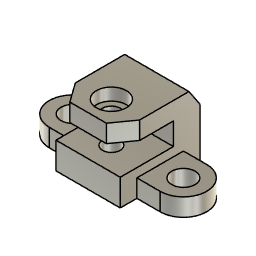
exercise05 (Autodesk Fusion 360 design; units mm, degrees)
Autodesk Fusion 360 part; units mm, degrees
sketch "草图1" plane through (0, 0, 0) normal (0, 0, 1) x (1, 0, 0)
  line L0 (-125, 0) -> (125, 0) construction
  line L1 (0, -50) -> (0, 50) construction
  line L2 (-58, 0) -> (58, 0)
  line L3 (58, 30) -> (58, 0)
  line L4 (58, 30) -> (100, 30)
  line L5 (-58, 0) -> (-58, 30)
  line L6 (-58, 30) -> (-100, 30)
  circle A0 centre (-100, 72) radius 21
  circle A1 centre (100, 72) radius 21
  circle A2 centre (0, 42) radius 16
  line L7 (-100, 114) -> (-58, 114)
  line L8 (-58, 114) -> (-58, 144)
  line L9 (-58, 144) -> (58, 144)
  line L10 (58, 144) -> (58, 114)
  line L11 (58, 114) -> (100, 114)
  arc A3 (100, 30) -> (100, 114) centre (100, 72) ccw
  arc A4 (-100, 114) -> (-100, 30) centre (-100, 72) ccw
  line L12 (-58, 114) -> (-58, 30)
  line L13 (58, 114) -> (58, 30)
  dimension "d1" = 116
  dimension "d2" = 144
  dimension "d3" = 72
  dimension "d4" = 200
  dimension "d5" = 84
  dimension "d6" = 42
  dimension "d7" = 32
  dimension "d8" = 42
  constraint horizontal L0
  constraint vertical L1
  constraint coincident L0 L2.start
  constraint coincident L0 L2.end
  constraint perpendicular L0 L3
  constraint perpendicular L3 L4
  constraint perpendicular L2 L5
  constraint perpendicular L5 L6
  constraint concentric A0 A4
  constraint concentric A1 A3
  constraint vertical L8
  constraint perpendicular L8 L9
  constraint perpendicular L8 L11
  constraint equal A3 A4
  constraint equal A0 A1
  constraint parallel L0 L7
  constraint perpendicular L9 L10
  constraint symmetric L1 L8 L10
  constraint symmetric L1 L3 L5
  constraint equal L3 L5
  constraint equal L8 L10
  constraint symmetric L1 A0.centre A1.centre
  constraint collinear L1.start L1.end A2.centre
  constraint tangent L4 A4
  constraint tangent L7 A4
  constraint collinear L5 L8
  measures "d1" distance of L2.start L2.end
  measures "d2" vertical distance of L2.end L9.end
  measures "d3" vertical distance of A1.centre L9.end
  measures "d4" distance of A0.centre A1.centre
  measures "d5" diameter of A3
  measures "d6" diameter of A1
  measures "d7" diameter of A2
  measures "d8" distance of L2 A2.centre
extrude "拉伸1" add sketch "草图1" along normal blind 32 contours L6 L7 A4 L12 | L4 L11 A3 L13 makes body 1 at (65, 72, 0) makes body 2 at (-65, 72, 0)
extrude "拉伸2" add sketch "草图1" along normal blind 48 contours L2 L3 L5 L8 L9 L10 L12 L13 bodies 1 2
sketch "草图2" plane through (-58, 0, 0) normal (-1, 0, 0) x (0, -1, 0)
  line L0 (-114, 0) -> (-114, 32)
  line L1 (-114, 32) -> (-30, 32)
  line L2 (-30, 32) -> (-30, 0)
  line L3 (-30, 0) -> (0, 0)
  line L4 (0, 0) -> (0, 48)
  line L5 (0, 48) -> (-144, 48)
  line L6 (-144, 48) -> (-144, 0)
  line L7 (-144, 0) -> (-114, 0)
  line L8 (-144, 48) -> (-144, 50)
  line L9 (-144, 50) -> (-144, 90)
  line L10 (-144, 90) -> (-124, 120)
  line L11 (-124, 120) -> (-96, 120)
  line L12 (-96, 120) -> (-96, 48)
  line L13 (-144, 48) -> (-96, 48)
  point P0 (-144, 0)
  dimension "d13" = 20
  dimension "d14" = 30
  dimension "d15" = 96
  dimension "d16" = 120
  constraint coincident L5.end L6.start
  constraint perpendicular L5 L8
  constraint perpendicular L5 L9
  constraint perpendicular L6 L11
  constraint coincident L5 L12.end
  constraint perpendicular L5 L12
  measures "d13" horizontal distance of L9.end L10.end
  measures "d14" vertical distance of L9.end L10.end
  measures "d15" distance of L4.end L12
  measures "d16" vertical distance of L10.end P0
extrude "拉伸3" add sketch "草图2" against normal blind 116 contours L5 L8 L9 L10 L11 L12 L13 bodies 1
sketch "草图3" plane through (0, 0, 120) normal (0, 0, 1) x (-1, 0, 0)
  line L0 (58, -124) -> (58, -96)
  line L1 (58, -96) -> (-58, -96)
  line L2 (-58, -96) -> (-58, -124)
  line L3 (-58, -124) -> (58, -124)
  line L4 (0, -180) -> (0, 50) construction
  line L5 (58, -96) -> (58, -35)
  line L6 (58, -35) -> (33, 0)
  line L7 (33, 0) -> (-33, 0)
  line L8 (-33, 0) -> (-58, -35)
  line L9 (-58, -35) -> (-58, -96)
  line L10 (58, -96) -> (-58, -96)
  circle A0 centre (0, -42) radius 27
  circle A1 centre (0, -42) radius 16
  line L11 (100, 0) -> (-125.4385, 0) construction
  dimension "d19" = 116
  dimension "d20" = 66
  dimension "d21" = 35
  dimension "d22" = 54
  dimension "d23" = 32
  dimension "d25" = 42
  constraint vertical L4
  constraint coincident L0.end L1.start
  constraint perpendicular L1 L5
  constraint perpendicular L5 L7
  constraint coincident L1.end L2.start
  constraint parallel L4 L9
  constraint symmetric L4 L6 L8
  constraint concentric A0 A1
  constraint collinear origin L4.end A0.centre
  constraint perpendicular L0 L11
  constraint collinear L7 L11
  constraint equal L5 L9
  measures "d19" distance of L0.end L1.end
  measures "d20" distance of L6.end L7.end
  measures "d21" distance of L7 L8.end
  measures "d22" diameter of A0
  measures "d23" diameter of A1
  measures "d25" distance of L7 A0.centre
extrude "拉伸4" add sketch "草图3" against normal blind 32 contours L1 L5 L6 L7 L8 L9 L10 | A0 bodies 1
extrude "拉伸5" cut sketch "草图3" against normal blind 22 contours A0 bodies 1
equation "d5 = ( 42 * 2 ) * 1 mm"
